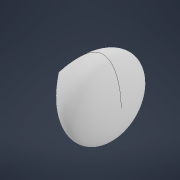
# Autodesk Inventor part: test spin toy bottom
Saved by Autodesk Inventor 2022 (Build 260153000, 153)
## iProperties
Created: 2021-05-31
Part Number: test spin toy bottom
Material: Generic
Document SubType Name: Modeling
Designer: sidsa
Density: 1 g/cm^3
Appearance: Default
Author: sidsa
## iProperties of the stored document test spin toy_3DPrint.ipt
Created: 2021-05-31
Part Number: test spin toy_3DPrint
Material: Generic
Document SubType Name: Modeling
Designer: sidsa
Density: 1 g/cm^3
Appearance: Default
Author: sidsa
Autodesk Inventor part; units mm, degrees
ref_plane "YZ Plane" through (0, 0, 0) normal (1, 0, 0) x (0, 1, 0)
ref_plane "XZ Plane" through (0, 0, 0) normal (0, 1, 0) x (-1, 0, 0)
ref_plane "XY Plane" through (0, 0, 0) normal (0, 0, 1) x (1, 0, 0)
sketch "Sketch1" plane through (0, 0, 0) normal (0, 0, 1) x (1, 0, 0)
  spline S0 degree 5 poles (0, 0) (1.6794, 2.0153) (3.359, 4.0308) (5.045, 6.0401) (8.3598, 9.9376) (11.7583, 13.7609) (13.4423, 15.5999) (16.701, 19.0191) (20.1453, 22.2559) (21.8214, 23.7259) (25.0365, 26.3061) (28.5489, 28.4419) (30.236, 29.2993) (33.7337, 30.596) (37.5009, 30.6259) (39.328, 30.1757) (46.3458, 26.1718) (48.9096, 17.582) (50.1746, 12.3101) (50.8057, 5.9191) (50.8, 0) knots 0 0 0 0 0 0 0.153806 0.153806 0.153806 0.29993 0.29993 0.29993 0.430709 0.430709 0.430709 0.540808 0.540808 0.540808 0.647062 0.647062 0.647062 1 1 1 1 1 1
  line L0 (0, 0) -> (50.8, 0)
  constraints: 2 end point, 1 horizontal, 1 horizontal alignment, 2 other
revolve "Revolution1" add sketch "Sketch1" angle 360 about axis through (0, 0, 0) along (1, 0, 0)
equation "curve S0 of \"Sketch1\": x = t; y = 0.6 ul*t*sqrt(4 ul-t*t); t from d0 to d1"
body "Solid1"
